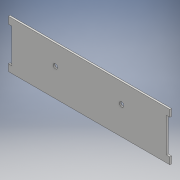
# Autodesk Inventor part: flipper-support
Saved by Autodesk Inventor 2017 (Build 210142000, 142)
## iProperties
Created: 2017-03-05
Part Number: flipper-support
Material: Generic
Document SubType Name: Modeling
Designer: John
Density: 1 g/cm^3
Appearance: Default
Author: John
Autodesk Inventor part; units mm, degrees
ref_plane "YZ Plane" through (0, 0, 0) normal (1, 0, 0) x (0, 1, 0)
ref_plane "XZ Plane" through (0, 0, 0) normal (0, 1, 0) x (-1, 0, 0)
ref_plane "XY Plane" through (0, 0, 0) normal (0, 0, 1) x (1, 0, 0)
sketch "Sketch1" plane through (0, 0, 0) normal (0, 1, 0) x (-1, 0, 0)
  line L0 (0, 0) -> (271, 0)
  line L1 (271, 0) -> (271, 84)
  line L2 (271, 84) -> (0, 84)
  line L3 (0, 84) -> (0, 0)
  line L4 (135.5, 84) -> (135.5, 0) construction
  line L5 (0, 84) -> (-6, 84)
  line L6 (-6, 84) -> (-6, 72)
  line L7 (-6, 72) -> (0, 72)
  line L8 (0, 72) -> (0, 84)
  line L9 (0, 0) -> (-6, 0)
  line L10 (-6, 0) -> (-6, 12)
  line L11 (-6, 12) -> (0, 12)
  line L12 (0, 12) -> (0, 0)
  line L13 (271, 84) -> (271, 0)
  line L14 (271, 84) -> (277, 84)
  line L15 (277, 84) -> (277, 72)
  line L16 (277, 72) -> (271, 72)
  line L17 (271, 72) -> (271, 84)
  line L18 (271, 0) -> (277, 0)
  line L19 (277, 0) -> (277, 12)
  line L20 (277, 12) -> (271, 12)
  line L21 (271, 12) -> (271, 0)
  circle A0 centre (194.5, 49.407) radius 4
  circle A1 centre (78.5, 49.407) radius 4
  line L22 (194.5, 49.407) -> (78.5, 49.407) construction
  dimension "d0" = 271
  dimension "d1" = 84
  dimension "d2" = 6
  dimension "d3" = 12
  dimension "d4" = 6
  dimension "d5" = 12
  dimension "d8" = 8
  dimension "d9" = 76.5
  dimension "d10" = 8
  dimension "d11" = 116
  dimension "d13" = 34.593
  constraints: 46 end point, 6 parallel, 6 symmetric about line, 4 horizontal, 3 perpendicular, 2 centre point, 2 midpoint
  measures "d0" distance of L2.end L1.end
  measures "d1" distance of L1.end L0.end
  measures "d2" distance of L7.end L6.end
  measures "d3" distance of L6.end L5.end
  measures "d4" distance of L10.end L11.end
  measures "d5" distance of L9.end L10.end
  measures "d8" diameter of A0
  measures "d9" distance from line of L1 L22.start
  measures "d10" diameter of A1
  measures "d11" distance of L22.end L22.start
  measures "d13" distance from line of L2 L22.start
extrude "Extrusion1" add sketch "Sketch1" along normal blind 3
body "Solid1"
